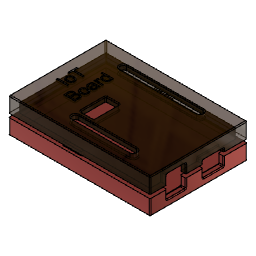
Board - Carlos Martin Parra (Autodesk Fusion 360 design; units mm, degrees)
Autodesk Fusion 360 part; units mm, degrees
box "BoxPrimitive1" add length 46.99 width 71.12 height 11 placed x (0, 1, 0) y (-1, 0, 0) z (0, 0, 1) at (71.12, 0, 0) makes body 1
shell "Shell1" thickness 3 outward yes removed faces 0 bodies 1
sketch "Sketch4" plane through (74.12, 0, 0) normal (1, 0, 0) x (0, 1, 0)
  line L0 (-3, 14) -> (-3, -3)
  line L1 (-3, -3) -> (49.99, -3)
  line L2 (49.99, -3) -> (49.99, 14)
  line L3 (49.99, 14) -> (-3, 14)
  line L4 (16.4809, 0.5202) -> (6.0809, 0.5202)
  line L5 (6.0809, 0.5202) -> (6.0809, 10.5202)
  line L6 (6.0809, 10.5202) -> (16.4809, 10.5202)
  line L7 (16.4809, 10.5202) -> (16.4809, 0.5202)
  line L8 (25.7874, 0.7529) -> (37.1874, 0.7529)
  line L9 (37.1874, 0.7529) -> (37.1874, 7.2529)
  line L10 (37.1874, 7.2529) -> (25.7874, 7.2529)
  line L11 (25.7874, 7.2529) -> (25.7874, 0.7529)
extrude "Extrude1" cut sketch "Sketch4" against normal blind 5 contours L4 L5 L6 L7 | L8 L9 L10 L11 bodies 1
sketch "Sketch5" plane through (0, 0, 14) normal (0, 0, 1) x (-1, 0, 0)
  line L0 (-74.12, -49.99) -> (3, -49.99)
  line L1 (3, -49.99) -> (3, 3)
  line L2 (3, 3) -> (-74.12, 3)
  line L3 (-74.12, 3) -> (-74.12, -49.99)
sketch "Sketch6" plane through (0, 0, 14) normal (0, 0, 1) x (-1, 0, 0)
  line L0 (-24, -9) -> (-31.4, -9)
  line L1 (-31.4, -9) -> (-31.4, -22.9)
  line L2 (-31.4, -22.9) -> (-24, -22.9)
  line L3 (-24, -22.9) -> (-24, -9)
extrude "Extrude2" cut sketch "Sketch6" against normal blind 5 bodies 1
fillet "Fillet1" radius 0.47 4 faces at (73.12, 13.0142, 0.5202) (73.12, 16.4809, 7.1869) (72.12, 9.5475, 10.5202) (73.12, 6.0809, 3.8536) on bodies 1
fillet "Fillet2" radius 0.47 4 faces at (73.12, 29.5874, 0.7529) (72.12, 25.7874, 2.9195) (73.12, 33.3874, 7.2529) (72.12, 37.1874, 5.0862) on bodies 1
fillet "Fillet3" radius 0.47 4 faces at (24, 18.2667, 13) (28.9333, 22.9, 13) (31.4, 13.6333, 13) (26.4667, 9, 13) on bodies 1
sketch "Sketch7" plane through (0, 0, 14) normal (0, 0, 1) x (-1, 0, 0)
  line L0 (-15.0011, -39.6977) -> (-56.7011, -39.6977)
  arc A0 (-56.7011, -39.6977) -> (-56.7011, -43.2477) centre (-56.7011, -41.4727) ccw
  line L1 (-56.7011, -43.2477) -> (-15.0011, -43.2477)
  arc A1 (-15.0011, -43.2477) -> (-15.0011, -39.6977) centre (-15.0011, -41.4727) ccw
  line L2 (-15.0011, -41.4727) -> (-56.7011, -41.4727) construction
  line L3 (-25.4504, -3.2055) -> (-56.9504, -3.2055)
  arc A2 (-56.9504, -3.2055) -> (-56.9504, -6.7555) centre (-56.9504, -4.9805) ccw
  line L4 (-56.9504, -6.7555) -> (-25.4504, -6.7555)
  arc A3 (-25.4504, -6.7555) -> (-25.4504, -3.2055) centre (-25.4504, -4.9805) ccw
  line L5 (-25.4504, -4.9805) -> (-56.9504, -4.9805) construction
  dimension "d30" = 41.7
  dimension "d31" = 3.55
  dimension "d32" = 3.55
  constraint tangent L0 A0
  constraint tangent A0 L1
  constraint parallel L0 L1
  constraint tangent L1 A1
  constraint tangent L0 A1
  constraint horizontal L2
  constraint tangent L3 A2
  constraint tangent A2 L4
  constraint parallel L3 L4
  constraint tangent L4 A3
  constraint tangent L3 A3
  constraint horizontal L5
  measures "d30" distance of A1.centre A0.centre
  measures "d31" diameter of A0
  measures "d32" diameter of A2
extrude "Extrude3" cut sketch "Sketch7" against normal blind 5 bodies 1
fillet "Fillet4" radius 0.47 8 faces at (28.9011, 39.6977, 13) (13.3832, 42.2028, 12) (42.8011, 43.2477, 13) (58.4098, 41.9535, 12) (46.4504, 6.7555, 13) (58.0914, 6.3403, 13) (35.9504, 3.2055, 13) (25.0124, 3.2604, 13) on bodies 1
fillet "Fillet5" radius 0.5 104 faces at (48.5072, 22.9611, 14) (28.9011, 39.4139, 13.9616) (58.808, 42.1806, 13.9995) (42.8011, 43.5068, 13.95) (14.1378, 43.5208, 13.9995) (13.3832, 42.2028, 12.1567) (28.9011, 39.6977, 12.8433) (58.4098, 41.9535, 12.1567) (42.8011, 43.2477, 12.8433) (42.8011, 43.5829, 11.0197) (13.9381, 39.5208, 11.0005) (28.9011, 39.4387, 11.05) (57.4613, 43.5613, 11.0005) (48.5072, 22.9611, 11) (23.8059, 23.0632, 11.0005) (28.7767, 23.2163, 11.0258) (31.5632, 23.0941, 11.0005) (31.6953, 13.79, 11.0337) (31.5941, 8.8368, 11.0005) (26.6233, 8.5524, 11.0005) (23.6753, 9.0112, 11.0005) (24.3163, 9.0258, 12.8433) (24, 18.11, 12.8433) (23.7047, 18.11, 13.9663) (23.8059, 23.0632, 13.9995) (24.0337, 22.6047, 12.8433) (28.7767, 22.9, 12.8433) (31.3742, 22.5837, 12.8433) (31.4, 13.79, 12.8433) (31.0837, 9.0258, 12.8433) (26.6233, 9, 12.8433) (26.6233, 8.5747, 13.9979) (23.8059, 8.8368, 13.9995) (31.0172, 8.5565, 13.9995) (31.7163, 13.79, 13.9742) (31.5632, 23.0941, 13.9995) (28.7767, 23.1953, 13.9663) (23.6837, 18.11, 11.0258) (46.4504, 6.8185, 11.235) (58.9764, 4.0664, 11.0005) (35.9504, 3.1797, 11.3163) (23.245, 5.2569, 11.0005) (25.0124, 3.2604, 12.8433) (23.245, 5.2569, 13.9995) (46.4504, 6.7561, 13.5524) (46.4504, 6.7555, 12.8433) (58.0914, 6.3403, 12.1567) (58.9764, 4.0664, 13.9995) (35.9504, 3.205, 13.5524) (35.9504, 3.2055, 12.8433) (48.4133, -3, 2.6667) (74.12, 45.8791, 5.9276) (74.1195, 5.6498, 0.8166) (72.2767, 6.3159, 0.5832) (71.1205, 5.7352, 0.5697) (71.12, 43.8791, 5.9276) (71.4153, 9.7042, 0.4866) (71.1205, 16.7322, 0.423) (72.9633, 16.2459, 0.5832) (72.9633, 12.8575, 0.5202) (73.8037, 12.8575, 0.4944) (74.1195, 16.9244, 0.903) (73.8247, 16.5145, 7.0302) (74.1195, 16.675, 10.6835) (72.9633, 16.1856, 10.4866) (71.1205, 16.675, 10.6835) (71.4153, 16.5145, 4.0102) (72.9633, 16.4809, 7.0302) (71.4153, 12.8575, 10.5539) (71.4576, 6.4356, 10.5255) (72.9633, 6.1438, 10.2852) (72.2767, 9.7042, 10.5202) (73.8037, 9.7042, 10.5461) (74.1195, 6.1304, 10.8658) (73.8037, 6.055, 4.0102) (72.9633, 6.0809, 4.0102) (71.4153, 6.0472, 7.0302) (71.1205, 26.1702, 0.3094) (72.9633, 26.0827, 0.7865) (72.9633, 25.7874, 4.9295) (72.9633, 26.0827, 7.2192) (71.1205, 25.7986, 7.5776) (71.4153, 29.744, 7.2865) (71.1205, 37.6091, 6.9992) (71.4153, 37.221, 4.9295) (71.1205, 37.5845, 0.9227) (71.4153, 33.2307, 0.7192) (72.9633, 29.744, 0.7529) (73.8247, 29.744, 0.7192) (74.1195, 26.1702, 0.3094) (73.8037, 25.7615, 4.9295) (74.1195, 25.7986, 7.5776) (73.8247, 33.2307, 7.2865) (74.1195, 37.6091, 6.9992) (72.9633, 36.9524, 7.1899) (72.9633, 37.1874, 3.0762) (72.9633, 36.9524, 0.8158) (74.1195, 37.6091, 1.0065) (73.8037, 37.2132, 3.0762) (72.9633, 33.2307, 7.2529) (71.4153, 25.7537, 3.0762) (48.4133, 49.99, 2.6667) (-3, 32.3267, 2.6667) (22.7067, 14.6633, -3) on bodies 1
ref_plane "WorkPlane1" through (35.56, 23.495, 5.5) normal (0, 0, -1) x (0, -1, 0)
split "Split1" by plane through (35.56, 23.495, 5.5) normal (0, 0, -1) bodies 1 makes body 2 at (22.8733, 14.83, -3)
copy_body "Body->Comp1" bodies 1 removing the originals makes body 3 in component "Component"
copy_body "Body->Comp2" bodies 2 removing the originals makes body 4 in component "Component'"
sketch "Sketch8" plane through (0, 0, 14) normal (0, 0, 1) x (-1, 0, 0)
  line L0 (-25, 0, -8.5) -> (-35, 0, -8.5)
  line L1 (-35, 0, -8.5) -> (-35, 1.5, -8.5)
  line L2 (-35, 1.5, -8.5) -> (-25, 1.5, -8.5)
  line L3 (-25, 1.5, -8.5) -> (-25, 0, -8.5)
  line L4 (-35, -47.0089, -8.5) -> (-25, -47.0089, -8.5)
  line L5 (-25, -47.0089, -8.5) -> (-25, -48.5089, -8.5)
  line L6 (-25, -48.5089, -8.5) -> (-35, -48.5089, -8.5)
  line L7 (-35, -48.5089, -8.5) -> (-35, -47.0089, -8.5)
  dimension "d39" = 10
  dimension "d40" = 1.5
  dimension "d41" = 10
  dimension "d42" = 1.5
extrude "Extrude1'" add sketch "Sketch8" along normal blind 2 contours L0 L1 L2 L3 | L4 L5 L6 L7 in plane through (0, 0, 5.5) normal (0, 0, 1) bodies 4 in component "Component'"
move_body "Move1" bodies 3 to x (1, 0, 0) y (0, 1, 0) z (0, 0, 1) at (0, 0, 2) in component "Component"
sketch "Sketch9" plane through (0, 0, 16) normal (0, 0, 1) x (-1, 0, 0)
  line L0 (-25.4504, -7.2255) -> (-56.9504, -7.2255)
  arc A0 (-56.9504, -2.7355) -> (-56.9504, -7.2255) centre (-56.9504, -4.9805) ccw
  line L1 (-56.9504, -2.7355) -> (-25.4504, -2.7355)
  arc A1 (-25.4504, -7.2255) -> (-25.4504, -2.7355) centre (-25.4504, -4.9805) ccw
  arc A2 (-24.47, -23.37) -> (-23.53, -22.43) centre (-24.47, -22.43) ccw
  line L2 (-24.47, -23.37) -> (-30.93, -23.37)
  arc A3 (-31.87, -22.43) -> (-30.93, -23.37) centre (-30.93, -22.43) ccw
  line L3 (-31.87, -22.43) -> (-31.87, -9.47)
  arc A4 (-30.93, -8.53) -> (-31.87, -9.47) centre (-30.93, -9.47) ccw
  line L4 (-30.93, -8.53) -> (-24.47, -8.53)
  arc A5 (-23.53, -9.47) -> (-24.47, -8.53) centre (-24.47, -9.47) ccw
  line L5 (-23.53, -9.47) -> (-23.53, -22.43)
  line L6 (-56.7011, -39.2277) -> (-15.0011, -39.2277)
  arc A6 (-15.0011, -43.7177) -> (-15.0011, -39.2277) centre (-15.0011, -41.4727) ccw
  line L7 (-15.0011, -43.7177) -> (-56.7011, -43.7177)
  arc A7 (-56.7011, -39.2277) -> (-56.7011, -43.7177) centre (-56.7011, -41.4727) ccw
  line L8 (-73.62, -49.49) -> (2.5, -49.49)
  line L9 (2.5, -49.49) -> (2.5, 2.5)
  line L10 (2.5, 2.5) -> (-73.62, 2.5)
  line L11 (-73.62, 2.5) -> (-73.62, -49.49)
  line L12 (-17.1074, -14.0213) -> (-17.1074, -31.5548) construction
  line L13 (-17.1074, -31.5548) -> (-2.4019, -31.5548) construction
  line L14 (-2.4019, -31.5548) -> (-2.4019, -14.0213) construction
  line L15 (-2.4019, -14.0213) -> (-17.1074, -14.0213) construction
  text T0 "IoT\nBoard" font "Arial" height 6 align centre top in box 17.5335 x 14.7055 at (-17.1074, -14.0213) x (0, -1) y (1, 0) spacing 1 kerned
extrude "Extrude1''" cut sketch "Sketch9" against normal blind 1 text T0 bodies 3 in component "Component"
component "Component" placed x (1, 0, 0) y (0, 1, 0) z (0, 0, 1) at (0, 0, 0)
component "Component'" placed x (1, 0, 0) y (0, 1, 0) z (0, 0, 1) at (0, 0, 0)
